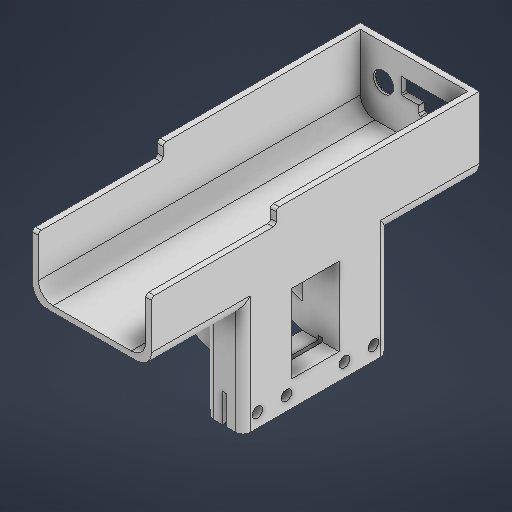
# Autodesk Inventor part: Copy of Revised Battery and Rotation Sensor Holder
Saved by Autodesk Inventor 2025.1 (Build 291241020, 241B)
## iProperties
Created: 2024-12-11
Part Number: Copy of Revised Battery and Rotation Sensor Holder
Material: Generic
Document SubType Name: Modeling
Designer: AtuStem
Density: 1 g/cm^3
Appearance: Default
Author: AtuStem
Autodesk Inventor part; units mm, degrees
ref_plane "YZ Plane" through (0, 0, 0) normal (1, 0, 0) x (0, 1, 0)
ref_plane "XZ Plane" through (0, 0, 0) normal (0, 1, 0) x (-1, 0, 0)
ref_plane "XY Plane" through (0, 0, 0) normal (0, 0, 1) x (1, 0, 0)
sketch "Sketch1" plane through (0, 0, 0) normal (1, 0, 0) x (0, 1, 0)
  line L0 (0, 0) -> (0, -12.7)
  circle A0 centre (0, -12.7) radius 3.9624
  line L1 (-6.096, -31.75) -> (5.08, -31.75)
  line L2 (5.08, -31.75) -> (5.08, 0)
  line L3 (5.08, 0) -> (-6.096, 0)
  line L4 (-6.096, 0) -> (-6.096, -31.75)
  circle A1 centre (0, -25.4) radius 3.9624
  line L5 (5.08, -10.3505) -> (41.91, -10.3505)
  line L6 (41.91, -10.3505) -> (41.91, -31.75)
  line L7 (41.91, -31.75) -> (5.08, -31.75)
  line L8 (5.08, -31.75) -> (5.08, -10.3505)
  line L9 (41.91, -71.755) -> (39.37, -71.755)
  line L10 (39.37, -71.755) -> (39.37, 0)
  line L11 (39.37, 0) -> (41.91, 0)
  line L12 (41.91, 0) -> (41.91, -71.755)
  line L13 (0, 0) -> (0, 12.7)
  circle A2 centre (0, 12.7) radius 3.9624
  line L14 (-6.096, 31.75) -> (5.08, 31.75)
  line L15 (5.08, 31.75) -> (5.08, 0)
  line L16 (-6.096, 0) -> (-6.096, 31.75)
  circle A3 centre (0, 25.4) radius 3.9624
  line L17 (5.08, 10.3505) -> (41.91, 10.3505)
  line L18 (41.91, 10.3505) -> (41.91, 31.75)
  line L19 (41.91, 31.75) -> (5.08, 31.75)
  line L20 (5.08, 31.75) -> (5.08, 10.3505)
  line L21 (41.91, 71.755) -> (39.37, 71.755)
  line L22 (39.37, 71.755) -> (39.37, 0)
  line L23 (41.91, 0) -> (41.91, 71.755)
  circle A4 centre (0, -25.4) radius 2.286
  circle A5 centre (0, -12.7) radius 2.286
  circle A6 centre (0, 12.7) radius 2.286
  circle A7 centre (0, 25.4) radius 2.286
  point P0 (39.37, -31.75)
  point P1 (39.37, -10.3505)
  point P2 (39.37, 10.3505)
  point P3 (39.37, 31.75)
  point P4 (40.64, 0)
  point P5 (40.64, -71.755)
  dimension "d0" = 12.7
  dimension "d1" = 7.9248
  dimension "d3" = 6.096
  dimension "d4" = 5.08
  dimension "d5" = 7.9248
  dimension "d6" = 12.7
  dimension "d7" = 6.35
  dimension "d8" = 10.3505
  dimension "d9" = 36.83
  dimension "d11" = 2.54
  dimension "d31" = 4.572
  dimension "d32" = 4.572
  dimension "d33" = 4.572
  dimension "d34" = 4.572
  dimension "d46" = 71.755
  dimension "d47" = 0
  dimension "d96" = 34.29
  constraints: 48 end point, 11 symmetric about line, 8 centre point, 6 coincident, 6 parallel, 3 horizontal, 3 perpendicular, 2 midpoint, 2 point on line, 1 vertical, 2 other
  measures "d0" distance of L0.start L0.end
  measures "d1" diameter of A0
  measures "d3" distance from line of L4 L0.end
  measures "d4" distance from line of L2 L0.end
  measures "d5" diameter of A1
  measures "d6" distance of A1.centre L0.end
  measures "d7" distance from line of L1 A1.centre
  measures "d8" distance between parallel lines of L3 L5
  measures "d9" distance of L5.start L5.end
  measures "d11" distance of L9.start L9.end
  measures "d31" diameter of A4
  measures "d32" diameter of A6
  measures "d33" diameter of A7
  measures "d34" diameter of A5
  measures "d46" distance of point (40.64, 0) point (40.64, -71.755)
  measures "d47" distance between parallel lines of L3 L11
  measures "d96" distance between parallel lines of L8 L10
extrude "Extrusion1" add sketch "Sketch1" along normal blind 16.2306 contours A0 | L4 L3 L2 L1 | L2 L5 L10 L7 | L16 L14 L15 L3 | L19 L22 L17 L15 | A1 | A2 | A3 | A4 | A5 | A6 | A7
extrude "Extrusion2" add sketch "Sketch1" along normal blind 16.2306 and the other way blind 35.814 contours L10 L5 L6 L7 | L7 L12 L9 L10 | L10 L11 L12 L5 | L22 L17 L23 L11 | L22 L21 L23 L19 | L19 L18 L17 L22
extrude "Extrusion3" cut sketch "Sketch1" along normal blind 2.54 contours A0 | A1 | A2 | A3 | A4 | A5 | A6 | A7
extrude "Extrusion4" cut sketch "Sketch1" along normal up to surface (16.2306 mm away) contours A4 | A5 | A6 | A7
sketch "Sketch3" plane through (0, -6.096, 31.75) normal (0, 0, 1) x (1, 0, 0)
  line L0 (0, 0) -> (16.2306, 0) projected
  line L1 (7.2644, 0) -> (8.9662, 0)
  line L2 (8.9662, 0) -> (8.9662, 12.7)
  line L3 (8.9662, 12.7) -> (7.2644, 12.7)
  line L4 (7.2644, 12.7) -> (7.2644, 0)
  line L5 (16.2306, 45.466) -> (16.2306, 0) projected
  line L6 (0, 45.466) -> (0, 0) projected
  point P0 (0, 6.096)
  dimension "d37" = 1.7018
  dimension "d38" = 12.7
  dimension "d39" = 16.2306
  dimension "d40" = 7.2644
  dimension "d41" = 7.2644
  constraints: 8 end point, 2 parallel, 1 horizontal, 1 perpendicular, 1 point on line
  measures "d37" distance between parallel lines of L2 L4
  measures "d38" distance of L1.end L2.end
  measures "d39" distance between parallel lines of L5 L6
  measures "d40" distance between parallel lines of L5 L2
  measures "d41" distance between parallel lines of L4 L6
extrude "Extrusion5" cut sketch "Sketch3" against normal up to surface (63.5 mm away)
sketch "Sketch4" plane through (-35.814, 41.91, 71.755) normal (0, 1, 0) x (1, 0, 0)
  line L0 (0, 143.51) -> (0, 0) projected
  line L1 (52.0446, 143.51) -> (0, 143.51)
  line L2 (0, 143.51) -> (0, 140.97)
  line L3 (0, 140.97) -> (52.0446, 140.97)
  line L4 (52.0446, 140.97) -> (52.0446, 143.51)
  line L5 (0, 0) -> (52.0446, 0) projected
  line L6 (0, 143.51) -> (2.54, 143.51)
  line L7 (2.54, 143.51) -> (2.54, 0)
  line L8 (2.54, 0) -> (0, 0)
  line L9 (0, 0) -> (0, 143.51)
  line L10 (52.0446, 143.51) -> (49.5046, 143.51)
  line L11 (49.5046, 143.51) -> (49.5046, 0)
  line L12 (49.5046, 0) -> (52.0446, 0)
  line L13 (52.0446, 0) -> (52.0446, 143.51)
  point P0 (35.814, 71.755)
  point P1 (49.5046, 140.97)
  point P2 (2.54, 140.97)
  dimension "d48" = 2.54
  dimension "d51" = 2.54
  dimension "d52" = 2.54
  constraints: 24 end point, 6 parallel, 3 horizontal, 3 perpendicular, 3 point on line
  measures "d48" distance between parallel lines of L3 L1
  measures "d51" distance between parallel lines of L7 L0
  measures "d52" distance between parallel lines of L13 L11
extrude "Extrusion6" add sketch "Sketch4" along normal blind 31.115 contours L1 L7 L3 L0 | L3 L7 L5 L0 | L1 L11 L3 L7 | L1 L4 L3 L11 | L3 L13 L5 L11
fillet "Fillet2" radius 6.35 1 edges at (-33.274, 41.91, 1.27)
fillet "Fillet3" radius 6.35 1 edges at (13.6906, 41.91, 1.27)
sketch "Sketch5" plane through (16.2306, 73.025, -71.755) normal (0, 0, -1) x (-1, 0, 0)
  circle A0 centre (39.4178, -14.9911) radius 4.445
  circle A1 centre (39.4178, -14.9911) radius 6.0325
  line L0 (23.1678, -19.7179) -> (16.5278, -19.7179)
  ellipse E0 centre (23.1678, -18.9677) end of major axis (23.1678, -19.7179) minor radius 0.75 (23.1678, -19.7179) -> (23.9178, -18.9677) ccw
  line L1 (23.9178, -16.0582) -> (23.9178, -18.9677)
  line L2 (31.2478, -15.9566) -> (24.0194, -15.9566)
  line L3 (31.7478, -9.3143) -> (31.7478, -15.4565)
  line L4 (8.4478, -8.8142) -> (31.2478, -8.8142)
  line L5 (7.9478, -15.4565) -> (7.9478, -9.3143)
  line L6 (15.6762, -15.9566) -> (8.4478, -15.9566)
  line L7 (15.7778, -18.9677) -> (15.7778, -16.0582)
  ellipse E1 centre (16.5278, -18.9677) end of major axis (16.5278, -19.7179) minor radius 0.75 (15.7778, -18.9677) -> (16.5278, -19.7179) ccw
  ellipse E2 centre (31.2478, -15.4565) end of major axis (31.2478, -15.9566) minor radius 0.5 (31.2478, -15.9566) -> (31.7478, -15.4565) ccw
  ellipse E3 centre (31.2478, -9.3143) end of major axis (31.2478, -9.8145) minor radius 0.5 (31.7478, -9.3143) -> (31.2478, -8.8142) ccw
  ellipse E4 centre (8.4478, -9.3143) end of major axis (8.4478, -9.8145) minor radius 0.5 (8.4478, -8.8142) -> (7.9478, -9.3143) ccw
  ellipse E5 centre (8.4478, -15.4565) end of major axis (8.4478, -15.9566) minor radius 0.5 (7.9478, -15.4565) -> (8.4478, -15.9566) ccw
  arc A2 (15.7778, -16.0582) -> (15.6762, -15.9566) centre (15.6762, -16.0582) ccw
  arc A3 (24.0194, -15.9566) -> (23.9178, -16.0582) centre (24.0194, -16.0582) ccw
  constraints: 16 end point, 4 centre point, 4 point on circle, 4 tangent, 1 equal radius, 24 other
extrude "Extrusion7" cut sketch "Sketch5" against normal up to surface (2.54 mm away) contours A0 | L0 E1 L7 A2 L6 E5 L5 E4 L4 E3 L3 E2 L2 A3 L1 E0
chamfer "Chamfer1" distance 1.5875 angle 45 1 edges at (-18.7422, 58.0339, -71.755)
sketch "Sketch10" plane through (-35.814, 0, 0) normal (-1, 0, 0) x (0, 0, 1)
  line L0 (71.755, 48.26) -> (71.755, 73.025) projected
  line L1 (71.755, 73.025) -> (17.145, 73.025)
  line L2 (17.145, 73.025) -> (17.145, 66.7258)
  line L3 (17.145, 66.7258) -> (71.755, 66.7258)
  line L4 (71.755, 66.7258) -> (71.755, 73.025)
  line L5 (-71.755, 39.37) -> (-71.755, 73.025) projected
  point P0 (0, 0)
  point P1 (-71.755, 45.72)
  dimension "d91" = 6.2992
  dimension "d92" = 88.9
  constraints: 8 end point, 2 parallel, 1 horizontal, 1 perpendicular
  measures "d91" distance of L1.end L2.end
  measures "d92" distance between parallel lines of L2 L5
extrude "Extrusion11" cut sketch "Sketch10" against normal up to surface (52.0446 mm away)
fillet "Fillet8" radius 1.27 6 edges at (-34.544, 73.025, 17.145) (-34.544, 66.7258, 17.145) (14.9606, 73.025, 17.145) (14.9606, 66.7258, 17.145) (-34.544, 66.7258, 71.755) (14.9606, 66.7258, 71.755)
sketch "Sketch11" plane through (0, 5.08, -10.3505) normal (0, 0, 1) x (1, 0, 0)
  line L0 (0, 34.29) -> (-17.5006, 34.29)
  line L1 (-17.5006, 34.29) -> (-17.5006, 0)
  line L2 (-17.5006, 0) -> (0, 0)
  line L3 (0, 0) -> (0, 34.29)
  line L4 (0, 0) -> (-17.5006, 0)
  line L5 (-17.5006, 0) -> (-17.5006, 12.7762)
  line L6 (0, 12.7762) -> (0, 0)
  circle A0 centre (-17.5006, 12.7762) radius 5.08
  circle A1 centre (-17.5006, 12.7762) radius 2.286
  line L7 (0, 0) -> (-19.4505, 8.0853)
  line L8 (-15.5507, 17.4671) -> (0, 11.0028)
  line L9 (-17.5006, 34.29) -> (-35.7574, 34.29)
  line L10 (-35.814, 34.29) -> (-35.814, 67.945) projected
  line L11 (-35.814, 34.29) -> (-21.8979, 10.2326)
  line L12 (-13.1033, 15.3198) -> (-24.0766, 34.29)
  line L13 (-35.814, 34.29) -> (16.2306, 34.29) projected
  point P0 (0, -5.08)
  point P1 (-20.7875, 16.6495)
  point P2 (-17.5006, 7.2748)
  point P3 (-17.5006, 7.6962)
  point P4 (-17.5006, 17.8562)
  point P5 (0, 11.0028)
  point P6 (-13.9638, 16.8074)
  dimension "d97" = 17.5006
  dimension "d100" = 10.16
  dimension "d101" = 4.572
  constraints: 24 end point, 5 point on circle, 3 parallel, 3 point on line, 3 tangent, 2 centre point, 2 coincident, 2 horizontal, 2 perpendicular
  measures "d97" distance between parallel lines of L1 L3
  measures "d100" diameter of A0
  measures "d101" diameter of A1
extrude "Extrusion12" add sketch "Sketch11" along normal blind 31.4325 and the other way blind 10.7061 contours L12 L8 A0 L1 | L1 A0 L11 L13 L9 L12 | L3 L7 L1 A0 L12 L8 | A0 L1 A1 | L1 A1 A0 | L12 A0 L8 | L7 A0 L1
sketch "Sketch12" plane through (0, 5.08, 10.3505) normal (1, 0, 0) x (0, 0, -1)
  line L0 (0, 34.29) -> (-21.3995, 34.29) projected
  line L1 (20.701, 0) -> (0, 0) projected
  line L2 (0, 34.29) -> (20.701, 34.29)
  line L3 (20.701, 34.29) -> (20.701, 0)
  line L4 (20.701, 0) -> (0, 0)
  line L5 (0, 0) -> (0, 34.29)
  point P0 (10.3505, -5.08)
  point P1 (-8.0264, 34.29)
  constraints: 8 end point, 2 parallel, 1 horizontal, 1 perpendicular
extrude "Extrusion13" cut sketch "Sketch12" against normal blind 28.7274
fillet "Fillet11" radius 3.175 5 edges at (0, 16.637, 31.75) (16.2306, 16.637, 31.75) (0, -6.096, 0) (0, 16.637, -31.75) (16.2306, 16.637, -31.75)
sketch "Sketch13" plane through (16.2306, 0, 0) normal (1, 0, 0) x (0, 0, -1)
  line L0 (-10.3505, 16.0828) -> (-10.3505, 39.37) projected
  line L1 (10.3505, 5.08) -> (-10.3505, 5.08) projected
  line L2 (-10.3505, 39.37) -> (10.3505, 39.37)
  line L3 (10.3505, 39.37) -> (10.3505, 5.08)
  line L4 (10.3505, 5.08) -> (-10.3505, 5.08)
  line L5 (-10.3505, 5.08) -> (-10.3505, 39.37)
  point P0 (0, 0)
  constraints: 8 end point, 2 parallel, 1 horizontal, 1 perpendicular
extrude "Extrusion14" cut sketch "Sketch13" against normal blind 63.5
fillet "Fillet13" radius 6.35 2 edges at (-13.9638, 21.8874, 15.7163) (-13.9638, 21.8874, -15.7035)
fillet "Fillet14" radius 6.35 5 edges at (16.2306, 39.37, 50.165) (16.2306, 39.37, -50.165) (-35.814, 39.37, 46.4185) (-35.814, 39.37, -46.4058) (-35.814, 39.37, 0)
fillet "Fillet15" radius 6.35 2 edges at (-35.814, 39.37, -15.7035) (-35.814, 39.37, 15.7163)
body "Solid1"
